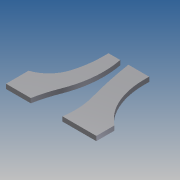
# Autodesk Inventor part: UA-70 Platten aussen
Saved by Autodesk Inventor 2014 (Build 180170000, 170)
## iProperties
Created: 2014-07-02
Part Number: UA-70 Platten aussen
Material: Allgemein
Document SubType Name: Modeling
Designer: Semenov
Density: 1 g/cm^3
Appearance: Vorgabe
Author: Semenov
Autodesk Inventor part; units mm, degrees
ref_plane "YZ Plane" through (0, 0, 0) normal (1, 0, 0) x (0, 1, 0)
ref_plane "XZ Plane" through (0, 0, 0) normal (0, 1, 0) x (-1, 0, 0)
ref_plane "XY Plane" through (0, 0, 0) normal (0, 0, 1) x (1, 0, 0)
sketch "Skizze3" plane through (0, 0, 0) normal (0, 0, 1) x (1, 0, 0)
  line L0 (-500, 500) -> (500, 500)
  line L1 (500, 500) -> (500, -500)
  line L2 (500, -500) -> (-500, -500)
  line L3 (-500, -500) -> (-500, 500)
  line L4 (-500, 500) -> (-275, 500)
  line L5 (-275, 500) -> (-275, 440)
  line L6 (-275, 440) -> (-500, 440)
  line L7 (-500, 440) -> (-500, 500)
  line L8 (500, 500) -> (275, 500)
  line L9 (275, 500) -> (275, 440)
  line L10 (275, 440) -> (500, 440)
  line L11 (500, 440) -> (500, 500)
  line L12 (-275, 500) -> (275, 500)
  line L13 (275, 500) -> (275, 300)
  line L14 (275, 300) -> (-275, 300)
  line L15 (-275, 300) -> (-275, 500)
  line L16 (-225, 300) -> (225, 300)
  line L17 (225, 300) -> (225, 360)
  line L18 (225, 360) -> (-225, 360)
  line L19 (-225, 360) -> (-225, 300)
  line L20 (-500, -500) -> (500, -500)
  line L21 (500, -500) -> (500, -440)
  line L22 (500, -440) -> (-500, -440)
  line L23 (-500, -440) -> (-500, -500)
  line L24 (-440, 440) -> (-500, 440)
  line L25 (-500, 440) -> (-500, -440)
  line L26 (-500, -440) -> (-440, -440)
  line L27 (-440, -440) -> (-440, 440)
  line L28 (500, 440) -> (440, 440)
  line L29 (440, 440) -> (440, -440)
  line L30 (440, -440) -> (500, -440)
  line L31 (500, -440) -> (500, 440)
  arc A0 (-270, -10) -> (-225, 300) centre (-1315.2778, 300) ccw
  arc A1 (-500, -250) -> (-270, -10) centre (-617.8721, 93.1691) ccw
  arc A2 (225, 300) -> (280, 0) centre (1070.6818, 300) ccw
  arc A3 (280, 0) -> (500, -300) centre (931.7592, 247.2901) ccw
  arc A4 (-150, -240) -> (-95, 360) centre (-1146.8979, 153.9031) ccw
  arc A5 (-150, -240) -> (-225, -500) centre (1170.154, -761.631) ccw
  arc A6 (-5, 360) -> (105, -150) centre (4524.0164, 1069.9839) ccw
  arc A7 (125, -500) -> (105, -150) centre (-696.9412, -371.3966) ccw
  circle A8 centre (-165, 430) radius 12.5
  circle A9 centre (-65, 430) radius 12.5
  circle A10 centre (115, 430) radius 12.5
  line L32 (-440, 440) -> (-500, 440)
  line L33 (-500, 440) -> (-500, -440)
  line L34 (-500, -440) -> (-440, -440)
  line L35 (-440, -440) -> (-440, 440)
  line L36 (440, -440) -> (500, -440)
  line L37 (500, -440) -> (500, 440)
  line L38 (500, 440) -> (440, 440)
  line L39 (440, 440) -> (440, -440)
  line L40 (-500, -250) -> (-500, -500)
  line L41 (-500, -500) -> (-225, -500)
  line L42 (-225, 360) -> (-95, 360)
  line L43 (-95, 360) -> (-5, 360)
  line L44 (-5, 360) -> (225, 360)
  line L45 (-225, -500) -> (125, -500)
  line L46 (125, -500) -> (500, -500)
  line L47 (500, -500) -> (500, -300)
  point P0 (0, 0)
  point P1 (-500.0625, 0)
  point P2 (0, 500.0625)
  point P3 (-500, 0)
  point P4 (0, 500)
  point P5 (0, 360)
  dimension "d5" = 1000
  dimension "d8" = 1000
  dimension "d9" = 60
  dimension "d10" = 225
  dimension "d11" = 225
  dimension "d12" = 550
  dimension "d13" = 200
  dimension "d14" = 450
  dimension "d15" = 60
  dimension "d16" = 60
  dimension "d17" = 880
  dimension "d18" = 60
  dimension "d19" = 60
  dimension "d20" = 250
  dimension "d21" = 230
  dimension "d22" = 240
  dimension "d23" = 200
  dimension "d24" = 300
  dimension "d25" = 220
  dimension "d26" = 130
  dimension "d27" = 150
  dimension "d28" = 275
  dimension "d29" = 75
  dimension "d30" = 260
  dimension "d31" = 90
  dimension "d32" = 230
  dimension "d33" = 375
  dimension "d34" = 350
  dimension "d35" = 365
  dimension "d36" = 350
  dimension "d37" = 20
  dimension "d38" = 25
  dimension "d39" = 70
  dimension "d40" = 60
  dimension "d41" = 110
  dimension "d42" = 30
  constraints: 96 end point, 22 parallel, 16 point on circle, 13 perpendicular, 11 centre point, 11 point on line, 10 horizontal, 6 tangent, 5 horizontal alignment, 3 collinear, 3 midpoint, 3 vertical alignment, 2 equal radius
  measures "d5" distance of L0.end L1.end
  measures "d8" distance of L0.start L0.end
  measures "d9" distance of L8.end L9.end
  measures "d10" distance of L9.end L10.end
  measures "d11" distance of L5.end L6.end
  measures "d12" distance of L13.end L14.end
  measures "d13" distance of L12.end L13.end
  measures "d14" distance of L17.end L18.end
  measures "d15" distance between parallel lines of L16 L18
  measures "d16" distance between parallel lines of L20 L22
  measures "d17" distance of L26.end L24.start
  measures "d18" distance between parallel lines of L25 L27
  measures "d19" distance between parallel lines of L29 L1
  measures "d20" distance from line of L40.start L20
  measures "d21" distance from line of A0.start L25
  measures "d22" vertical distance of A0.start L40.start
  measures "d23" distance from line of L47.end L20
  measures "d24" vertical distance of A2.end L47.end
  measures "d25" distance from line of A2.end L31
  measures "d26" distance from line of L42.end L19
  measures "d27" distance edge to line of A4 L19
  measures "d28" distance from line of L41.end L3
  measures "d29" horizontal distance of A4.start L41.end
  measures "d30" vertical distance of A4.start L41.end
  measures "d31" distance of L43.end L42.end
  measures "d32" distance from line of L43.end L17
  measures "d33" distance from line of L45.end L1
  measures "d34" distance of L45.end L41.end
  measures "d35" distance edge to line of A7 L1
  measures "d36" vertical distance of A6.end L45.end
  measures "d37" horizontal distance of A6.end L45.end
  measures "d38" diameter of A8
  measures "d39" distance from line of A8.centre L12
  measures "d40" distance from line of A8.centre L19
  measures "d41" distance from line of A10.centre L17
  measures "d42" horizontal distance of A9.centre L42.end
extrude "Extrusion9" add sketch "Skizze3" against normal blind 50 contours A1 L27 L22 L3 | L22 A5 L2 L3 | A1 A0 L14 A4 A5 L22 L27 | L19 L18 A4 L14 | L1 L22 L29 A3 | L29 L22 A7 A6 L14 A2 A3 | L14 A6 L18 L17 | L1 L2 A7 L22
equation "\"d16\" = d9"
equation "\"d18\" = d9"
equation "\"d19\" = d9"
